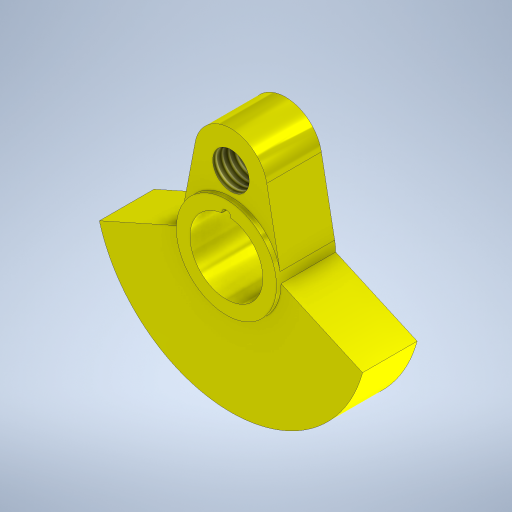
# Autodesk Inventor part: Crank
Saved by Autodesk Inventor 2023 (Build 270158000, 158)
## iProperties
Created: 2023-02-12
Part Number: Crank
Material: Iron, Cast
Document SubType Name: Modeling
Designer: NiveshandNisheeth
Density: 7.15 g/cm^3
Appearance: Iron - Cast
Author: NiveshandNisheeth
Autodesk Inventor part; units mm, degrees
ref_plane "YZ Plane" through (0, 0, 0) normal (1, 0, 0) x (0, 1, 0)
ref_plane "XZ Plane" through (0, 0, 0) normal (0, 1, 0) x (-1, 0, 0)
ref_plane "XY Plane" through (0, 0, 0) normal (0, 0, 1) x (1, 0, 0)
sketch "Sketch1" plane through (0, 0, 0) normal (0, 0, 1) x (1, 0, 0)
  line L0 (0, 17.4) -> (0, -20.4) construction
  line L1 (-20.2396, 0) -> (20.2396, 0) construction
  circle A0 centre (0, 0) radius 5.5
  circle A1 centre (0, 8) radius 2
  arc A2 (-14.4568, -4) -> (14.4568, -4) centre (0, 0) ccw
  line L2 (-14.4568, -4) -> (-5.5, 0)
  line L3 (5.5, 0) -> (14.4568, -4)
  line L4 (-3.9291, 8.7499) -> (-5.3921, 1.0839)
  line L5 (3.9291, 8.7499) -> (5.3921, 1.0839)
  arc A3 (3.9291, 8.7499) -> (-3.9291, 8.7499) centre (0, 8) ccw
  circle A4 centre (0, 0) radius 4
  arc A5 (5.3921, 1.0839) -> (-5.3921, 1.0839) centre (0, 0) ccw
  dimension "d0" = 11
  dimension "d1" = 4
  dimension "d3" = 8
  dimension "d4" = 15
  dimension "d5" = 4
  dimension "d6" = 8
  dimension "d7" = 21.61
  dimension "d8" = 4
  constraints: 9 point on circle, 8 end point, 6 centre point, 5 coincident, 3 point on line, 2 symmetric about line, 1 horizontal alignment, 1 tangent, 1 other
  measures "d0" diameter of A0
  measures "d1" diameter of A1
  measures "d3" distance of A0.centre A1.centre
  measures "d4" radius of A2
  measures "d5" vertical distance of L2.start L2.end
  measures "d6" diameter of A4
  measures "d7" angle of L5 L4
  measures "d8" radius of A3
extrude "Extrusion1" add sketch "Sketch1" along normal mid plane 6 contours L3 A2 L2 A0 | A0 L4 A3 L5
extrude "Extrusion2" add sketch "Sketch1" along normal blind 3.5 contours A0
extrude "Extrusion3" add sketch "Sketch1" against normal up to surface (3 mm away) contours A0
sketch "Sketch2" plane through (0, 0, 3.5) normal (0, 0, 1) x (1, 0, 0)
  circle A0 centre (0, 0) radius 4 construction
  circle A1 centre (0, 0) radius 5.5 construction
  circle A2 centre (0, 4) radius 0.5
  dimension "d16" = 1
  constraints: 1 centre point, 1 vertical alignment, 1 other
  measures "d16" diameter of A2
extrude "Extrusion4" cut sketch "Sketch2" against normal through all
thread "Thread1" size "M4x0.7" class "6H" standard "ANSI Metric M Profile" full length
equation "\"d6\" = d3"
body "Solid1"
